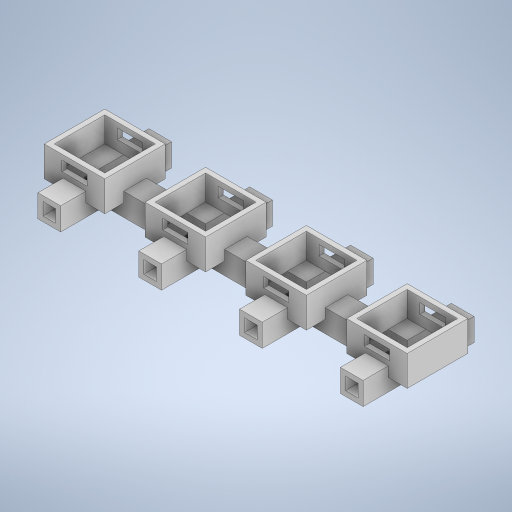
# Autodesk Inventor part: Part1
Saved by Autodesk Inventor 2023 (Build 270158000, 158)
## iProperties
Created: 2022-10-04
Part Number: Part1
Material: Generic
Document SubType Name: Modeling
Designer: Ty Gazaway
Density: 1 g/cm^3
Appearance: Default
Author: Ty Gazaway
Autodesk Inventor part; units mm, degrees
ref_plane "YZ Plane" through (0, 0, 0) normal (1, 0, 0) x (0, 1, 0)
ref_plane "XZ Plane" through (0, 0, 0) normal (0, 1, 0) x (-1, 0, 0)
ref_plane "XY Plane" through (0, 0, 0) normal (0, 0, 1) x (1, 0, 0)
sketch "Sketch1" plane through (0, 0, 0) normal (0, 1, 0) x (-1, 0, 0)
  line L0 (0, 0) -> (-79.375, 0)
  line L1 (-79.375, 0) -> (-79.375, -3.175)
  line L2 (-79.375, -3.175) -> (0, -3.175)
  line L3 (0, -3.175) -> (0, 0)
  line L4 (0, 11.1125) -> (-3.175, 11.1125)
  line L5 (-3.175, 11.1125) -> (-3.175, -14.2875)
  line L6 (-3.175, -14.2875) -> (0, -14.2875)
  line L7 (0, -14.2875) -> (0, 11.1125)
  line L8 (-25.4, -14.2875) -> (-25.4, 11.1125)
  line L9 (-25.4, 11.1125) -> (-28.575, 11.1125)
  line L10 (-28.575, 11.1125) -> (-28.575, -14.2875)
  line L11 (-28.575, -14.2875) -> (-25.4, -14.2875)
  line L12 (-50.8, -14.2875) -> (-50.8, 11.1125)
  line L13 (-50.8, 11.1125) -> (-53.975, 11.1125)
  line L14 (-53.975, 11.1125) -> (-53.975, -14.2875)
  line L15 (-53.975, -14.2875) -> (-50.8, -14.2875)
  line L16 (-76.2, -14.2875) -> (-76.2, 11.1125)
  line L17 (-76.2, 11.1125) -> (-79.375, 11.1125)
  line L18 (-79.375, 11.1125) -> (-79.375, -14.2875)
  line L19 (-79.375, -14.2875) -> (-76.2, -14.2875)
  point P0 (0, -1.5875)
  point P1 (0, -1.5875)
  point P2 (-1.5875, -14.2875)
  point P3 (-25.4, -1.5875)
  point P4 (-26.9875, -14.2875)
  point P5 (-50.8, -1.5875)
  point P6 (-52.3875, -14.2875)
  point P7 (-76.2, -1.5875)
  point P8 (-77.7875, -14.2875)
  point P9 (-1.5875, 11.1125)
  point P10 (-76.2, -3.175)
  point P11 (-79.375, -3.175)
  point P12 (-79.375, 0)
  point P13 (-76.2, 0)
  point P14 (-53.975, 0)
  point P15 (-50.8, 0)
  point P16 (-50.8, -3.175)
  point P17 (-53.975, -3.175)
  point P18 (-25.4, -3.175)
  point P19 (-28.575, -3.175)
  point P20 (-28.575, 0)
  point P21 (-25.4, 0)
  point P22 (-3.175, 0)
  point P23 (0, 0)
  point P24 (0, -3.175)
  point P25 (-3.175, -3.175)
  dimension "d0" = 79.375
  dimension "d1" = 3.175
  dimension "d20" = 3.175
  dimension "d25" = 25.4
  dimension "d31" = 12.7
  constraints: 40 end point, 4 midpoint, 4 parallel, 3 horizontal, 2 perpendicular, 1 coincident, 1 vertical alignment, 30 other
  measures "d0" distance of L2.end L1.end
  measures "d1" distance of L1.end L0.end
  measures "d20" distance of L6.end L5.end
  measures "d25" distance of L6.end L8.start
  measures "d31" vertical distance of point (0, -1.587) point (-1.588, 11.113)
extrude "Extrusion1" add sketch "Sketch1" along normal blind 3.175
sketch "Sketch2" plane through (0, 3.175, 0) normal (0, 1, 0) x (1, 0, 0)
  line L0 (-4.7625, -4.7625) -> (7.9375, -4.7625)
  line L1 (7.9375, -4.7625) -> (7.9375, 7.9375)
  line L2 (7.9375, 7.9375) -> (-4.7625, 7.9375)
  line L3 (-4.7625, 7.9375) -> (-4.7625, -4.7625)
  line L4 (0, 14.2875) -> (0, -11.1125) projected
  line L5 (20.6375, 7.9375) -> (20.6375, -4.7625)
  line L6 (20.6375, -4.7625) -> (33.3375, -4.7625)
  line L7 (33.3375, 7.9375) -> (20.6375, 7.9375)
  line L8 (33.3375, -4.7625) -> (33.3375, 7.9375)
  line L9 (46.0375, 7.9375) -> (46.0375, -4.7625)
  line L10 (46.0375, -4.7625) -> (58.7375, -4.7625)
  line L11 (58.7375, 7.9375) -> (46.0375, 7.9375)
  line L12 (58.7375, -4.7625) -> (58.7375, 7.9375)
  line L13 (71.4375, 7.9375) -> (71.4375, -4.7625)
  line L14 (71.4375, -4.7625) -> (84.1375, -4.7625)
  line L15 (84.1375, 7.9375) -> (71.4375, 7.9375)
  line L16 (84.1375, -4.7625) -> (84.1375, 7.9375)
  line L17 (3.175, 14.2875) -> (0, 14.2875) projected
  point P0 (-4.7625, 1.5875)
  point P1 (0, 1.5875)
  point P2 (0, 1.5875)
  point P3 (20.6375, 1.5875)
  point P4 (46.0375, 1.5875)
  point P5 (71.4375, 1.5875)
  point P6 (1.5875, 7.9375)
  point P7 (1.5875, 14.2875)
  dimension "d32" = 12.7
  dimension "d33" = 12.7
  dimension "d36" = 25.4
  constraints: 32 end point, 5 midpoint, 2 horizontal, 2 parallel, 1 collinear, 1 horizontal alignment, 1 perpendicular, 1 vertical alignment, 26 other
  measures "d32" distance of L2.end L1.end
  measures "d33" distance of L1.end L0.end
  measures "d36" distance of L2.end L5.start
extrude "Extrusion2" add sketch "Sketch2" along normal blind 6.35
shell "Shell2" thickness 1.27 outward yes removed faces 4 at (3.7042, 9.525, 0.5292) at (29.1042, 9.525, 0.5292) at (54.5042, 9.525, 0.5292) at (79.9042, 9.525, 0.5292)
sketch "Sketch3" plane through (4.445, -1.27, -15.5575) normal (0, 0, -1) x (-1, 0, 0)
  line L0 (4.445, 1.27) -> (4.445, 4.445) projected
  line L1 (1.27, 4.445) -> (4.445, 4.445) projected
  line L2 (1.27, 1.27) -> (1.27, 4.445) projected
  line L3 (1.27, 1.27) -> (4.445, 1.27) projected
  line L4 (4.445, 4.445) -> (1.27, 4.445) projected
  line L5 (4.445, 4.445) -> (1.27, 4.445)
  line L6 (1.27, 4.445) -> (1.27, 1.27)
  line L7 (1.27, 1.27) -> (4.445, 1.27)
  line L8 (4.445, 1.27) -> (4.445, 4.445)
  constraints: 8 end point, 2 parallel, 1 horizontal, 1 perpendicular
extrude "Extrusion3" cut sketch "Sketch3" against normal through all
pattern_linear "Rectangular Pattern1" count 4 spacing 25.4 along (1, 0, 0) of "Extrusion3"
sketch "Sketch4" plane through (34.6075, 1.905, -9.2075) normal (0, 0, -1) x (-1, 0, 0)
  line L0 (36.195, 6.35) -> (29.845, 6.35)
  line L1 (29.845, 6.35) -> (29.845, 3.81)
  line L2 (29.845, 3.81) -> (36.195, 3.81)
  line L3 (36.195, 3.81) -> (36.195, 6.35)
  line L4 (25.4, 7.62) -> (40.64, 7.62) projected
  point P0 (34.6075, -1.905)
  point P1 (33.02, 6.35)
  point P2 (33.02, 7.62)
  dimension "d47" = 6.35
  dimension "d48" = 2.54
  dimension "d49" = 1.27
  constraints: 8 end point, 2 midpoint, 2 parallel, 1 horizontal, 1 perpendicular, 1 vertical alignment
  measures "d47" distance of L2.end L1.end
  measures "d48" distance of L2.end L0.start
  measures "d49" distance between parallel lines of L4 L0
extrude "Extrusion4" cut sketch "Sketch4" against normal through all
pattern_linear "Rectangular Pattern2" count 4 spacing 25.4 along (1, 0, 0) of "Extrusion4"
body "Solid1"
